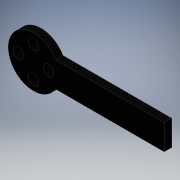
# Autodesk Inventor part: GripperLeftBar
Saved by Autodesk Inventor 2016 (Build 200138000, 138)
## iProperties
Created: 2016-03-31
Part Number: GripperLeftBar
Material: UHMW, Black
Document SubType Name: Modeling
Designer: mkepler
Density: 0.94 g/cm^3
Appearance: Smooth - Black
Mass: 1.91296 g
Surface Area: 19.6201 cm^2
Volume: 2.03507 cm^3
Author: mkepler
Autodesk Inventor part; units mm, degrees
ref_plane "YZ Plane" through (0, 0, 0) normal (1, 0, 0) x (0, 1, 0)
ref_plane "XZ Plane" through (0, 0, 0) normal (0, 1, 0) x (-1, 0, 0)
ref_plane "XY Plane" through (0, 0, 0) normal (0, 0, 1) x (1, 0, 0)
sketch "Sketch1" plane through (0, 0, 0) normal (0, 1, 0) x (-1, 0, 0)
  arc A0 (-8.6603, -5) -> (-8.6603, 5) centre (0, 0) ccw
  circle A1 centre (6, 0) radius 2.125
  circle A2 centre (-6, 0) radius 2.125
  circle A3 centre (0, -6) radius 2.125
  circle A4 centre (0, 6) radius 2.125
  line L0 (6, 0) -> (6, -4)
  line L1 (-38.6603, -5) -> (-8.6603, -5)
  line L2 (-44.6603, 5) -> (-24.6603, 5) construction
  line L3 (-38.6603, -5) -> (-51.6603, -5)
  line L4 (-8.6603, 5) -> (-51.6603, 5)
  line L5 (-51.6603, 5) -> (-51.6603, -5)
  dimension "d0" = 20
  dimension "d1" = 4.25
  dimension "d2" = 6
  dimension "d3" = 4.25
  dimension "d4" = 6
  dimension "d5" = 4.25
  dimension "d6" = 6
  dimension "d7" = 4.25
  dimension "d8" = 6
  dimension "d9" = 4
  dimension "d26" = 43
  dimension "d28" = 43
  constraints: 12 end point, 5 centre point, 3 horizontal, 3 point on circle, 1 coincident, 1 perpendicular, 1 vertical
  measures "d0" diameter of A0
  measures "d1" diameter of A1
  measures "d2" distance of point (0, 0) L0.start
  measures "d3" diameter of A2
  measures "d4" distance of point (0, 0) A2.centre
  measures "d5" diameter of A3
  measures "d6" distance of point (0, 0) A3.centre
  measures "d7" diameter of A4
  measures "d8" distance of point (0, 0) A4.centre
  measures "d9" distance of L0.start L0.end
  measures "d26" distance of L3.end L1.end
  measures "d28" distance of L4.start L4.end
extrude "Extrusion1" add sketch "Sketch1" against normal blind 3
body "Solid1"
